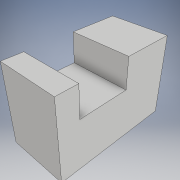
# Autodesk Inventor part: Part 2
Saved by Autodesk Inventor 2017.1 (Build 211199000, 199)
## iProperties
Created: 2016-10-22
Part Number: Part 2
Material: Generic
Document SubType Name: Modeling
Designer: rbibby53
Density: 1 g/cm^3
Appearance: Default
Author: rbibby53
Autodesk Inventor part; units mm, degrees
ref_plane "YZ Plane" through (0, 0, 0) normal (1, 0, 0) x (0, 1, 0)
ref_plane "XZ Plane" through (0, 0, 0) normal (0, 1, 0) x (-1, 0, 0)
ref_plane "XY Plane" through (0, 0, 0) normal (0, 0, 1) x (1, 0, 0)
sketch "Sketch1" plane through (0, 0, 0) normal (1, 0, 0) x (0, 1, 0)
  point P0 (0, 0)
sketch "Sketch2" plane through (0, 0, 0) normal (1, 0, 0) x (0, 1, 0)
  line L0 (12.2052, 5.8608) -> (-2.7948, 5.8608)
  line L1 (-2.7948, 5.8608) -> (-2.7948, -4.1392)
  line L2 (-2.7948, -4.1392) -> (12.2052, -4.1392)
  line L3 (12.2052, -4.1392) -> (12.2052, 5.8608)
  point P0 (0, 0)
  dimension "d0" = 15
  dimension "d1" = 10
  constraints: 8 end point, 2 parallel, 1 horizontal, 1 perpendicular
  measures "d0" distance of L1.end L2.end
  measures "d1" distance of L0.end L1.end
extrude "Extrusion1" add sketch "Sketch2" along normal blind 30
sketch "Sketch3" plane through (30, 0, 0) normal (1, 0, 0) x (0, 0, -1)
  line L0 (-5.8608, -2.7948) -> (4.1392, -2.7948) projected
  line L1 (-5.8608, -2.7948) -> (54.1392, -2.7948)
  line L2 (54.1392, -2.7948) -> (54.1392, -27.7948)
  line L3 (54.1392, -27.7948) -> (-5.8608, -27.7948)
  line L4 (-5.8608, -27.7948) -> (-5.8608, -2.7948)
  point P0 (0, 0)
  dimension "d4" = 60
  dimension "d5" = 25
  constraints: 8 end point, 2 parallel, 1 horizontal, 1 perpendicular
  measures "d4" distance of L2.end L3.end
  measures "d5" distance of L1.end L2.end
extrude "Extrusion2" add sketch "Sketch3" against normal blind 30
sketch "Sketch4" plane through (30, 0, 0) normal (1, 0, 0) x (0, 0, -1)
  line L0 (54.1392, -2.7948) -> (54.1392, -27.7948) projected
  line L1 (54.1392, -2.7948) -> (29.1392, -2.7948)
  line L2 (29.1392, -2.7948) -> (29.1392, 12.2052)
  line L3 (29.1392, 12.2052) -> (54.1392, 12.2052)
  line L4 (54.1392, 12.2052) -> (54.1392, -2.7948)
  point P0 (0, 0)
  dimension "d8" = 25
  dimension "d9" = 15
  constraints: 8 end point, 2 parallel, 1 horizontal, 1 perpendicular
  measures "d8" distance of L2.end L3.end
  measures "d9" distance of L1.end L2.end
extrude "Extrusion3" add sketch "Sketch4" against normal blind 30
sketch "Sketch5" plane through (30, -27.7948, -54.1392) normal (0, 0, -1) x (-1, 0, 0)
  line L0 (0, 0) -> (30, 0) projected
  line L1 (0, 0) -> (0, 5)
  line L2 (0, 40) -> (0, 0) projected
  line L3 (0, 5) -> (3, 5)
  line L4 (3, 5) -> (18, 5)
  line L5 (18, 5) -> (18, 15)
  line L6 (18, 15) -> (3, 15)
  line L7 (3, 15) -> (3, 5)
  point P0 (30, 27.7948)
  dimension "d12" = 5
  dimension "d13" = 3
  dimension "d14" = 15
  dimension "d15" = 10
  constraints: 12 end point, 2 parallel, 2 perpendicular, 1 horizontal, 1 point on line
  measures "d12" distance of L0.start L1.end
  measures "d13" distance of L1.end L3.end
  measures "d14" distance of L6.end L5.end
  measures "d15" distance of L4.end L5.end
extrude "Extrusion4" cut sketch "Sketch5" against normal blind 25
body "Solid1"
